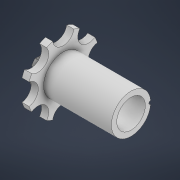
# Autodesk Inventor part: Part5
Saved by Autodesk Inventor 2021 (Build 250183000, 183)
## iProperties
Created: 2022-03-09
Part Number: Part5
Material: Generic
Document SubType Name: Modeling
Designer: ragv1
Density: 1 g/cm^3
Appearance: Default
Author: ragv1
Autodesk Inventor part; units mm, degrees
sketch "Sketch1" plane through (0, 0, 0) normal (1, 0, 0) x (0, 1, 0)
  circle A0 centre (0, 0) radius 5.5
  dimension "d1" = 11
  constraints: 1 centre point, 1 coincident
  measures "d1" diameter of A0
extrude "Extrusion1" add sketch "Sketch1" against normal blind 21.5
sketch "Sketch2" plane through (0, 0, 0) normal (1, 0, 0) x (0, 0, -1)
  circle A0 centre (0, 0) radius 4
  dimension "d4" = 8
  constraints: 1 centre point, 1 coincident
  measures "d4" diameter of A0
extrude "Extrusion2" cut sketch "Sketch2" against normal blind 12
sketch "Sketch3" plane through (-12, 0, 0) normal (1, 0, 0) x (0, 0, -1)
  circle A0 centre (0, 0) radius 2.5
  dimension "d7" = 5
  constraints: 1 centre point, 1 coincident
  measures "d7" diameter of A0
extrude "Extrusion3" cut sketch "Sketch3" against normal up to next
sketch "Sketch4" plane through (0, 0, 0) normal (1, 0, 0) x (0, 0, -1)
  arc A0 (5.4773, 0.4995) -> (5.4773, -0.4995) centre (5.5, 0) ccw
  circle A1 centre (0, 0) radius 2.5 projected
  arc A2 (5.4773, -0.4995) -> (5.4773, 0.4995) centre (0, 0) ccw
  dimension "d10" = 1
  dimension "d11" = 0
  dimension "d12" = 5.5
  dimension "d13" = 11
  constraints: 4 point on circle, 2 centre point, 1 coincident
  measures "d10" diameter of A0
  measures "d11" vertical distance of A1.centre A0.centre
  measures "d12" distance of A1.centre A0.centre
  measures "d13" diameter of A2
extrude "Extrusion4" cut sketch "Sketch4" against normal blind 15 contours A2 A0
ref_plane "Work Plane1" through (-21, 0, 0) normal (-1, 0, 0) x (0, 0, 1)
sketch "Sketch5" plane through (-21, 0, 0) normal (-1, 0, 0) x (0, 0, 1)
  arc A0 (-8.8502, 4.6555) -> (-4.6555, 8.8502) centre (-7.071, 7.071) ccw
  circle A1 centre (0, 0) radius 2.5 projected
  circle A2 centre (0, 0) radius 5.5
  arc A3 (-9.55, -2.9661) -> (-9.55, 2.9661) centre (-9.9999, 0) ccw
  arc A4 (-4.6555, -8.8502) -> (-8.8502, -4.6555) centre (-7.071, -7.071) ccw
  arc A5 (2.9661, -9.55) -> (-2.9661, -9.55) centre (0, -9.9999) ccw
  arc A6 (8.8502, -4.6555) -> (4.6555, -8.8502) centre (7.071, -7.071) ccw
  arc A7 (9.55, 2.9661) -> (9.55, -2.9661) centre (9.9999, 0) ccw
  arc A8 (4.6555, 8.8502) -> (8.8502, 4.6555) centre (7.071, 7.071) ccw
  arc A9 (-2.9661, 9.55) -> (2.9661, 9.55) centre (0, 9.9999) ccw
  arc A10 (-9.55, -2.9661) -> (-8.8502, -4.6555) centre (0, 0) ccw
  arc A11 (-4.6555, -8.8502) -> (-2.9661, -9.55) centre (0, 0) ccw
  arc A12 (2.9661, -9.55) -> (4.6555, -8.8502) centre (0, 0) ccw
  arc A13 (8.8502, -4.6555) -> (9.55, -2.9661) centre (0, 0) ccw
  arc A14 (9.55, 2.9661) -> (8.8502, 4.6555) centre (0, 0) ccw
  arc A15 (-2.9661, 9.55) -> (-4.6555, 8.8502) centre (0, 0) ccw
  arc A16 (4.6555, 8.8502) -> (2.9661, 9.55) centre (0, 0) ccw
  arc A17 (-2.9661, 9.55) -> (-4.6555, 8.8502) centre (0, 0) ccw
  arc A18 (-8.8502, 4.6555) -> (-9.55, 2.9661) centre (0, 0) ccw
  arc A19 (-9.55, -2.9661) -> (-8.8502, -4.6555) centre (0, 0) ccw
  arc A20 (-4.6555, -8.8502) -> (-2.9661, -9.55) centre (0, 0) ccw
  arc A21 (2.9661, -9.55) -> (4.6555, -8.8502) centre (0, 0) ccw
  arc A22 (8.8502, -4.6555) -> (9.55, -2.9661) centre (0, 0) ccw
  arc A23 (9.55, 2.9661) -> (8.8502, 4.6555) centre (0, 0) ccw
  arc A24 (4.6555, 8.8502) -> (2.9661, 9.55) centre (0, 0) ccw
  arc A25 (-2.9661, 9.55) -> (-4.6555, 8.8502) centre (0, 0) ccw
  dimension "d18" = 7.071
  dimension "d19" = 7.071
  dimension "d20" = 6
  dimension "d24" = 360
  dimension "d27" = 10
  dimension "d30" = 360
  constraints: 48 point on circle, 25 centre point, 4 coincident, 66 other
  measures "d18" horizontal distance of A1.centre A0.centre
  measures "d19" horizontal distance of A1.centre A0.centre
  measures "d20" diameter of A0
  measures "d27" radius of A18
extrude "Extrusion5" add sketch "Sketch5" against normal blind 2 contours A0 A15 A9 A16 A8 A14 A7 A13 A6 A12 A5 A11 A4 A10 A3 A18
ref_plane "Work Plane3" through (-21.5, 0, 0) normal (-1, 0, 0) x (0, 0, 1)
sketch "Sketch8" plane through (-21.5, 0, 0) normal (-1, 0, 0) x (0, 0, 1)
  line L0 (-2.5, 2.5) -> (-2.5, 4.899)
  line L1 (-2.5, 2.5) -> (-3.889, 3.889)
  arc A0 (-2.4999, 4.8989) -> (-3.889, 3.889) centre (0, 0) ccw
  point P0 (-2.5, 4.8988)
  dimension "d45" = 2.399
  dimension "d46" = 2.5
  dimension "d47" = 2.5
  dimension "d48" = 1.389
  dimension "d49" = 1.389
  constraints: 4 end point, 2 point on circle, 1 centre point, 1 coincident, 1 vertical
  measures "d45" distance of L0.start L0.end
  measures "d46" horizontal distance of point (0, 0) L0.start
  measures "d47" horizontal distance of point (0, 0) L0.start
  measures "d48" horizontal distance of L0.start L1.end
  measures "d49" horizontal distance of L0.start L1.end
extrude "Extrusion7" add sketch "Sketch8" along normal blind 1.5
pattern_circular "Circular Pattern1" count 8 over 360 about axis through (-12, 0, 0) along (-1, 0, 0) of "Extrusion7"
ref_plane "Work Plane4" through (-23, 0, -5.4999) normal (0.8575, 0.5145, 0) x (0, 0, 1)
sketch "Sketch9" plane through (-23, 0, -5.4999) normal (0.8575, 0.5145, 0) x (0, 0, 1)
  line L0 (0, 0) -> (1.9643, 0) projected
  line L1 (0, 0) -> (0.601, 2.9155)
  line L2 (0.601, 2.9155) -> (2.9999, 2.9155) projected
  line L3 (0, 0) -> (1.9643, 0)
  ellipse E0 centre (5.4999, 4.116) end of major axis (-0.0001, 4.116) minor radius 4.7162 (0.0226, 4.5443) -> (0.0226, 3.6877) ccw projected
  line L4 (0.601, 2.9155) -> (2.9999, 2.9155)
  ellipse E1 centre (5.4999, 0.7717) end of major axis (-0.0001, 0.7717) minor radius 4.7162 projected
  ellipse E2 centre (5.4999, 0.7717) end of major axis (2.9999, 0.7717) minor radius 2.1437 projected
  line L5 (2.9999, 2.9155) -> (3.2384, 1.6856)
  line L6 (1.9643, 0.7717) -> (1.9643, 0) projected
  line L7 (1.9643, 0) -> (3.2384, 1.6856)
  point P0 (5.4999, 11.8334)
  point P1 (0.2681, -1.4545)
  point P2 (0.0408, 0.1977)
  point P3 (0.074, 0)
  point P4 (0.074, 0)
  dimension "d69" = 1.2741
  constraints: 10 end point, 2 horizontal, 4 other
  measures "d69" horizontal distance of L0.end L5.end
extrude "Extrusion8" add sketch "Sketch9" along normal up to next contours E1 L1 L2 L5 L7 L0
pattern_circular "Circular Pattern2" count 8 over 360 about axis through (-12, 0, 0) along (-1, 0, 0) of "Extrusion8"
body "Solid1"
